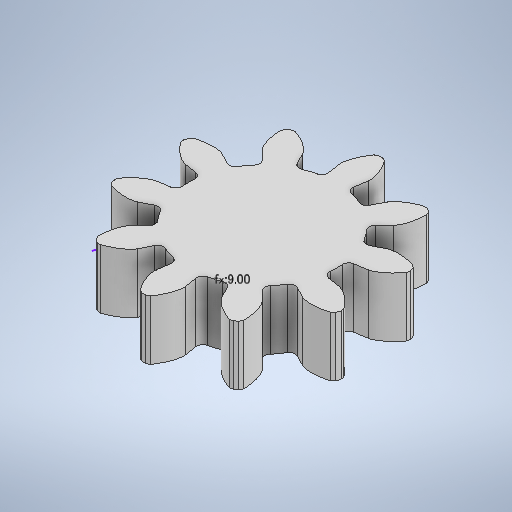
# Autodesk Inventor part: gear1
Saved by Autodesk Inventor 2025.2 (Build 292293000, 293)
## iProperties
Created: 2025-01-11
Part Number: gear1
Material: 一般
Document SubType Name: Modeling
Designer: mahhy
Density: 1 g/cm^3
Appearance: 既定
Author: mahhy
Autodesk Inventor part; units mm, degrees
ref_plane "YZ Plane" through (0, 0, 0) normal (1, 0, 0) x (0, 1, 0)
ref_plane "XZ Plane" through (0, 0, 0) normal (0, 1, 0) x (-1, 0, 0)
ref_plane "XY Plane" through (0, 0, 0) normal (0, 0, 1) x (1, 0, 0)
sketch "スケッチ2" plane through (0, 0, 0) normal (0, 1, 0) x (-1, 0, 0)
  line L0 (0, 0) -> (4.6406, 0.735)
  line L1 (0, 0) -> (4.6406, 0.735)
  line L2 (0, 0) -> (4.6985, 0) construction
  dimension "d13" = 9
  constraints: 6 end point, 1 collinear, 1 equal length, 1 horizontal, 4 other
  measures "d13" angle of L2 L1
sketch "スケッチ3" plane through (0, 0, 0) normal (0, 1, 0) x (-1, 0, 0)
  circle A0 centre (0, 0) radius 6
  dimension "d14" = 12
  constraints: 1 centre point, 1 coincident
  measures "d14" diameter of A0
extrude "押し出し1" add sketch "スケッチ3" along normal blind 3
sketch "スケッチ4" plane through (0, 3, 0) normal (0, 1, 0) x (1, 0, 0)
  spline S0 degree 3 poles (-4.6406, -0.735) (-4.6407, -0.735) (-5.0482, -0.8157) (-5.543, -1.3768) (-5.7641, -1.6276) (-5.9965, -1.9703) (-6.1909, -2.4132) knots 0 0 0 0 0.691133 0.691133 0.691133 1 1 1 1 projected
  line L0 (0, 0) -> (-4.6406, -0.735) projected
  line L1 (0, 0) -> (-6, 0)
  circle A0 centre (0, 0) radius 6 projected
  circle A1 centre (0, 0) radius 3.75
  point P0 (-3.7038, -0.5866)
  point P1 (-3.75, 0)
  point P2 (-5.7662, -1.6587)
  dimension "d17" = 7.5
  constraints: 2 end point, 1 centre point, 1 coincident, 1 horizontal, 2 other
  measures "d17" diameter of A1
extrude "押し出し2" cut sketch "スケッチ4" against normal blind 3 contours S0 A0 L1 A1 L0 picked at (-4.7969, -0.245)
fillet "フィレット1" radius 0.3 1 edges at (-3.7038, 1.5, 0.5866)
chamfer "面取り1" distance 0.1 angle 45 1 edges at (-5.7662, 1.5, 1.6587)
mirror "ミラー1" about plane through (-6, 3, 0) normal (0, 0, 1) of "押し出し2", "フィレット1", "面取り1"
pattern_circular "円形状パターン1" count 10 over 360 about axis through (0, -10, 0) along (0, 1, 0) of "押し出し2", "フィレット1", "面取り1", "ミラー1"
equation "\"module\" = 1"
